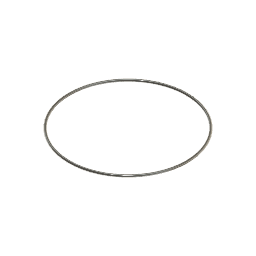
Challenger Seal v1 (Autodesk Fusion 360 design; units mm, degrees)
Autodesk Fusion 360 part; units mm, degrees
sketch "Sketch1" plane through (0, 0, 0) normal (0, 0, 1) x (1, 0, 0)
  circle A0 centre (0, 0) radius 54
  dimension "d1" = 108
  constraint coincident A0.centre origin
  measures "d1" diameter of A0
sketch "Sketch2" plane through (0, 0, 0) normal (1, 0, 0) x (0, 1, 0)
  circle A0 centre (54, 0) radius 1
  line L0 (54, 0) -> (-54, 0)
  dimension "d2" = 2
  dimension "d4" = 54
  constraint horizontal A0.centre origin
  measures "d2" diameter of A0
  measures "d4" distance of A0.centre origin
revolve "Revolve1" add sketch "Sketch2" angle 360 about axis through (0, 0, 1.75) along (0, 0, 1)
